Autodesk Fusion 360 part; units mm, degrees
note: some values were not read from the file. Set by a fixed rule: the direction of a hole.
(part 8 of 8)
  line L919 (41.979, -64.443) -> (42.137, -64.6279)
  line L920 (42.137, -64.6279) -> (42.2641, -64.8353)
  line L921 (42.2641, -64.8353) -> (42.3571, -65.06)
  line L922 (42.3571, -65.06) -> (42.4139, -65.2965)
  line L923 (42.4139, -65.2965) -> (42.433, -65.539)
  line L924 (42.433, -65.539) -> (42.4139, -65.7815)
  line L925 (42.4139, -65.7815) -> (42.3571, -66.018)
  line L926 (42.3571, -66.018) -> (42.2641, -66.2427)
  line L927 (42.2641, -66.2427) -> (42.137, -66.4501)
  line L928 (42.137, -66.4501) -> (41.979, -66.635)
  line L929 (41.979, -66.635) -> (41.7941, -66.793)
  line L930 (41.7941, -66.793) -> (41.5867, -66.9201)
  line L931 (41.5867, -66.9201) -> (41.362, -67.0131)
  line L932 (41.362, -67.0131) -> (41.1255, -67.0699)
  line L933 (41.1255, -67.0699) -> (40.883, -67.089)
  line L934 (40.883, -67.089) -> (40.6405, -67.0699)
  line L935 (40.6405, -67.0699) -> (40.404, -67.0131)
  line L936 (40.404, -67.0131) -> (40.1793, -66.9201)
  line L937 (40.1793, -66.9201) -> (39.9719, -66.793)
  line L938 (39.9719, -66.793) -> (39.787, -66.635)
  line L939 (39.787, -66.635) -> (39.629, -66.4501)
  line L940 (39.629, -66.4501) -> (39.5019, -66.2427)
  line L941 (39.5019, -66.2427) -> (39.4089, -66.018)
  line L942 (39.4089, -66.018) -> (39.3521, -65.7815)
  line L943 (39.3521, -65.7815) -> (39.333, -65.539)
  line L944 (39.333, -65.539) -> (39.3358, -65.5035)
  line L945 (39.3358, -65.5035) -> (39.3521, -65.2965)
  line L946 (39.3521, -65.2965) -> (39.4089, -65.06)
  line L947 (39.4946, -65.9741) -> (39.5843, -66.195)
  line L948 (39.5843, -66.195) -> (39.7089, -66.3983)
  line L949 (39.7089, -66.3983) -> (39.865, -66.5785)
  line L950 (39.865, -66.5785) -> (40.0485, -66.7308)
  line L951 (40.0485, -66.7308) -> (40.2543, -66.8511)
  line L952 (40.2543, -66.8511) -> (40.4771, -66.9362)
  line L953 (40.4771, -66.9362) -> (40.7107, -66.9837)
  line L954 (40.7107, -66.9837) -> (40.949, -66.9925)
  line L955 (40.949, -66.9925) -> (41.1855, -66.9622)
  line L956 (41.1855, -66.9622) -> (41.4139, -66.8937)
  line L957 (41.4139, -66.8937) -> (41.628, -66.7888)
  line L958 (41.628, -66.7888) -> (41.8221, -66.6503)
  line L959 (41.8221, -66.6503) -> (41.991, -66.482)
  line L960 (41.991, -66.482) -> (42.1302, -66.2884)
  line L961 (42.1302, -66.2884) -> (42.2358, -66.0746)
  line L962 (42.2358, -66.0746) -> (42.3051, -65.8465)
  line L963 (42.3051, -65.8465) -> (42.3362, -65.6101)
  line L964 (42.3362, -65.6101) -> (42.338, -65.539)
  line L965 (42.338, -65.539) -> (42.3184, -65.3014)
  line L966 (42.3184, -65.3014) -> (42.2603, -65.0701)
  line L967 (42.2603, -65.0701) -> (42.1653, -64.8515)
  line L968 (42.1653, -64.8515) -> (42.0358, -64.6513)
  line L969 (42.0358, -64.6513) -> (41.8753, -64.4749)
  line L970 (41.8753, -64.4749) -> (41.6882, -64.3271)
  line L971 (41.6882, -64.3271) -> (41.4794, -64.2119)
  line L972 (41.4794, -64.2119) -> (41.2547, -64.1323)
  line L973 (41.2547, -64.1323) -> (41.0199, -64.0905)
  line L974 (41.0199, -64.0905) -> (40.7815, -64.0876)
  line L975 (40.7815, -64.0876) -> (40.5458, -64.1236)
  line L976 (40.5458, -64.1236) -> (40.3192, -64.1977)
  line L977 (40.3192, -64.1977) -> (40.1077, -64.3078)
  line L978 (40.1077, -64.3078) -> (39.917, -64.451)
  line L979 (39.917, -64.451) -> (39.7523, -64.6234)
  line L980 (39.7523, -64.6234) -> (39.6179, -64.8203)
  line L981 (39.6179, -64.8203) -> (39.5175, -65.0366)
  line L982 (39.5175, -65.0366) -> (39.4538, -65.2664)
  line L983 (39.4538, -65.2664) -> (39.4285, -65.5035)
  line L984 (39.4285, -65.5035) -> (39.4422, -65.7415)
  line L985 (39.4422, -65.7415) -> (39.4946, -65.9741)
extrude "Extrude1" add sketch "SOLDERBREAD02_DXF_Outline_in_MilliMeters" along normal blind 2.54 contours L411 L412 L413 L414 L415 L416 L417 L418 L419 L420 L421 L422 L423 L424 L425 L426 L427 L428 L429 L430 L433 L434 L435 L436 L437 L440 L443 L444 L445 L446 L447 L450 L451 L452 L453 L454 L455 L456 L457 L458 L459 L460 L461 L462 L463 L464 L465 L466 L467 L468 L469 L470 L471 L472 L473 L474 L475 L476 L477 L478 L479 L480 L481 L482 L483 L484 L485 L486 L487 L488 L489 L490 L491 L492 L493 L494 L495 L496 L497 L498 L499 L500 L501 L502 L503 L504 L505 L506 L507 L508 L509 L510 L511 L512 L513 L514 L515 L516 L517 L518 L519 L520 L521 L523 L524 L525 L526 L527 L528 L529 L532 L533 L534 L535 L536 L537 L538 L539 L540 L541 L542 L543 L544 L545 L546 L547 L548 L549 L550 L551 L552 L553 L554 L555 L556 L557 L558 L559 L560 L561 L562 L563 L564 L565 L566 L567 L568 L569 L570 L571 L572 L573 L574 L575 L576 L577 L578 L579 L580 L581 L582 L583 L584 L585 L586 L587 L588 L589 L590 L591 L592 L593 L594 L595 L596 L599 L600 L601 L602 L603 L604 L605 L608 L609 L610 L611 L612 L616 L617 L618 L619 L620 L621 L622 L623 L624 L625 L626 L627 L628 L629 L630 L631 L632 L633 L634 L635 L636 L637 L638 L639 L640 L641 L642 L643 L644 L645 L646 L647 L648 L649 L650 L651 L652 L653 L654 L655 L656 L657 L658 L659 L660 L661 L662 L663 L664 L665 L666 L667 L668 L669 L670 L671 L672 L673 L674 L675 L676 L677 L678 L679 L680 L681 L682 L684 L685 L686 L687 L688 L689 L690 L691 L692 L693 L694 L695 L696 L697 L700 L701 L702 L703 L704 L705 L706 L707 L708 L709 L710 L711 L712 L713 L714 L715 L716 L717 L718 L719 L720 L721 L722 L723 L724 L725 L726 L727 L728 L729 L730 L731 L732 L733 L734 L735 L736 L737 L738 L739 L740 L741 L742 L743 L744 L745
